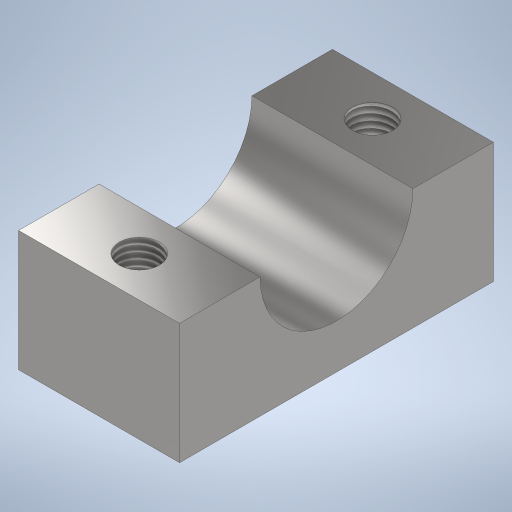
# Autodesk Inventor part: Clamp
Saved by Autodesk Inventor 2024 (Build 280153020, 153B)
## iProperties
Created: 2023-08-30
Part Number: Clamp
Material: Steel, Mild
Document SubType Name: Modeling
Designer: Victoria
Density: 7.85 g/cm^3
Appearance: Semi-Polished
Author: Victoria
Autodesk Inventor part; units mm, degrees
ref_plane "YZ Plane" through (0, 0, 0) normal (1, 0, 0) x (0, 1, 0)
ref_plane "XZ Plane" through (0, 0, 0) normal (0, 1, 0) x (-1, 0, 0)
ref_plane "XY Plane" through (0, 0, 0) normal (0, 0, 1) x (1, 0, 0)
sketch "Sketch1" plane through (0, 0, 0) normal (1, 0, 0) x (0, 1, 0)
  circle A0 centre (0, 0) radius 9.5
  line L0 (0, 9.5) -> (0, 19.5)
  line L1 (0, 19.5) -> (-15, 19.5)
  line L2 (0, -9.5) -> (0, -19.5)
  line L3 (0, -19.5) -> (-15, -19.5)
  line L4 (-15, -19.5) -> (-15, 19.5)
  dimension "d0" = 19
  dimension "d1" = 10
  dimension "d2" = 15
  dimension "d3" = 10
  constraints: 10 end point, 3 perpendicular, 2 point on circle, 2 vertical, 1 centre point, 1 coincident
  measures "d0" diameter of A0
  measures "d1" distance of L0.start L0.end
  measures "d2" distance of L0.end L1.end
  measures "d3" distance of L2.start L2.end
extrude "Extrusion1" add sketch "Sketch1" along normal blind 20 contours A0 L2 L3 L4 L1 L0
sketch "Sketch2" plane through (0, 0, 19.5) normal (0, 1, 0) x (1, 0, 0)
  line L0 (0, 0) -> (0, 5)
  line L1 (0, 0) -> (0, 39) projected
  line L2 (0, 5) -> (10, 5)
  line L3 (20, 0) -> (20, 39) projected
  circle A0 centre (10, 5) radius 2.5
  point P0 (0, 19.5)
  dimension "d6" = 5
  dimension "d7" = 10
  dimension "d8" = 5
  constraints: 4 end point, 1 centre point, 1 coincident, 1 perpendicular, 1 point on line
  measures "d6" distance of L0.start L0.end
  measures "d7" distance of L0.end L2.end
  measures "d8" diameter of A0
extrude "Extrusion2" cut sketch "Sketch2" against normal through all
thread "Thread1" size "M5x0.8" class "6H" standard "ISO Metric profile" full length
mirror "Mirror2" about plane through (0, 0, 0) normal (0, 0, 1) of "Extrusion2"
body "Solid1"
